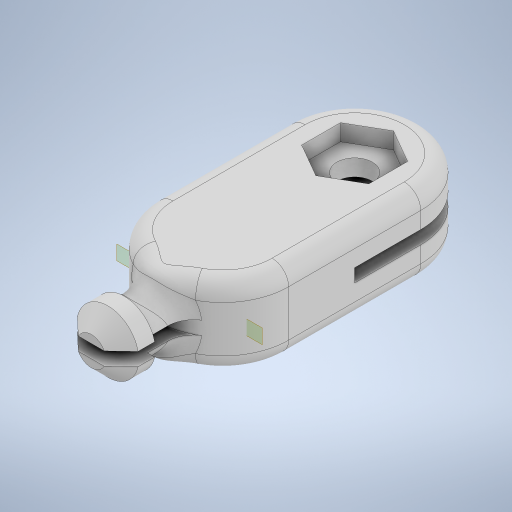
# Autodesk Inventor part: flipper_robot_v2_flipper_adapter
Saved by Autodesk Inventor 2023.1 (Build 271208000, 208)
## iProperties
Created: 2025-10-23
Part Number: flipper_robot_v2_flipper_adapter
Material: Generic
Document SubType Name: Modeling
Designer: Lars
Density: 1 g/cm^3
Appearance: Default
Author: Lars
Autodesk Inventor part; units mm, degrees
ref_plane "YZ Plane" through (0, 0, 0) normal (1, 0, 0) x (0, 1, 0)
ref_plane "XZ Plane" through (0, 0, 0) normal (0, 1, 0) x (-1, 0, 0)
ref_plane "XY Plane" through (0, 0, 0) normal (0, 0, 1) x (1, 0, 0)
sketch "Sketch1" plane through (0, 0, 0) normal (0, 1, 0) x (-1, 0, 0)
  line L0 (0, 4) -> (0, -4) construction
  line L1 (-4, 4) -> (-4, -4)
  line L2 (4, -4) -> (4, 4)
  arc A0 (4, 4) -> (-4, 4) centre (0, 4) ccw
  arc A1 (-4, -4) -> (4, -4) centre (0, -4) ccw
  circle A2 centre (0, -4) radius 1.075
  point P0 (0, 0)
  dimension "d0" = 4
  dimension "d1" = 8
  dimension "d2" = 2.15
  constraints: 8 end point, 4 point on circle, 4 tangent, 3 centre point, 1 coincident, 1 midpoint, 1 parallel, 1 vertical
  measures "d0" distance of point (0, 0) L0.end
  measures "d1" diameter of A1
  measures "d2" diameter of A2
extrude "Extrusion1" add sketch "Sketch1" along normal blind 2
sketch "Sketch2" plane through (0, 2, 0) normal (0, 1, 0) x (1, 0, 0)
  line L0 (-4, 4) -> (-4, -4) projected
  arc A0 (-4, -4) -> (4, -4) centre (0, -4) ccw projected
  line L1 (4, -4) -> (4, 4) projected
  line L2 (-4, 0) -> (4, 0)
  line L3 (0, 4) -> (0, -4) construction
  line L4 (-4, 0) -> (-4, -4)
  line L5 (4, -4) -> (4, 0)
  arc A1 (-4, -4) -> (4, -4) centre (0, -4) ccw
  point P0 (0, 0)
  constraints: 10 end point, 3 midpoint, 2 point on circle, 2 tangent, 1 centre point, 1 concentric, 1 parallel, 1 perpendicular
extrude "Extrusion2" add sketch "Sketch2" along normal blind 0.8
sketch "Sketch3" plane through (0, 2.8, 0) normal (0, 1, 0) x (1, 0, 0)
  line L0 (0, -4) -> (0, 4) construction
  line L1 (-4, -4) -> (-4, 4)
  line L2 (4, 4) -> (4, -4)
  arc A0 (-4, -4) -> (4, -4) centre (0, -4) ccw
  arc A1 (4, 4) -> (-4, 4) centre (0, 4) ccw
  circle A2 centre (0, 4) radius 1.075 projected
  circle A3 centre (0, 4) radius 1.075
  point P0 (0, 0)
  dimension "d7" = 4
  constraints: 8 end point, 4 point on circle, 4 tangent, 3 centre point, 1 coincident, 1 midpoint, 1 parallel, 1 vertical
  measures "d7" distance of point (0, 0) L0.end
extrude "Extrusion3" add sketch "Sketch3" along normal blind 2
ref_plane "Work Plane1" through (4, 2, 6) normal (0, 0, -1) x (-1, 0, 0)
sketch "Sketch4" plane through (4, 2, 6) normal (0, 0, -1) x (-1, 0, 0)
  line L0 (4, -2) -> (4, 2.8) construction
  line L1 (2.925, 2.8) -> (5.075, 2.8) projected
  line L2 (8, 0) -> (8, 0.8) projected
  line L3 (8, 0.4) -> (0, 0.4) construction
  circle A0 centre (4, 0.4) radius 2.4 construction
  line L4 (8, 2.8) -> (0, 2.8) projected
  line L5 (5.45, 0.8) -> (2.55, 0.8)
  line L6 (2.55, 0.8) -> (2.55, 0)
  line L7 (2.55, 0) -> (5.45, 0)
  line L8 (5.45, 0) -> (5.45, 0.8)
  circle A1 centre (4, 0.4) radius 1.45
  point P0 (5.45, 0.4)
  point P1 (2.55, 0.4)
  point P2 (2.0546, 1.8054)
  point P3 (5.041, 2.5625)
  point P4 (6.3869, 0.15)
  point P5 (1.6131, 0.15)
  point P6 (5.3937, 0)
  point P7 (2.6063, 0)
  point P8 (2.6063, 0.8)
  point P9 (5.3937, 0.8)
  dimension "d12" = 0.8
  dimension "d15" = 2.9
  dimension "d35" = 2.9
  constraints: 12 end point, 5 midpoint, 3 horizontal, 2 parallel, 2 point on circle, 1 centre point, 1 coincident, 1 perpendicular, 3 other
  measures "d12" distance of L6.end L5.end
  measures "d15" diameter of A1
  measures "d35" distance of L6.end L7.end
extrude "Extrusion4" add sketch "Sketch4" against normal blind 5.95 contours L5 A1 | A1 L7
sketch "Sketch6" plane through (4, 2, 11.95) normal (0, 0, 1) x (1, 0, 0)
  arc A0 (-2.1682, 0.8) -> (-5.8318, 0.8) centre (-4, 0.4) ccw
  line L0 (-5.3937, 0.8) -> (-5.8318, 0.8)
  arc A1 (-2.6063, 0.8) -> (-5.3937, 0.8) centre (-4, 0.4) ccw projected
  line L1 (-5.3937, 0.8) -> (-2.6063, 0.8) projected
  arc A2 (-2.6063, 0.8) -> (-5.3937, 0.8) centre (-4, 0.4) ccw projected
  line L2 (-5.3937, 0.8) -> (-2.6063, 0.8) projected
  line L3 (-2.6063, 0.8) -> (-2.1682, 0.8)
  line L4 (-5.8318, 0.8) -> (-5.3937, 0.8)
  point P0 (-4, -2)
  dimension "d16" = 3.75
  constraints: 6 end point, 2 collinear, 2 point on circle, 1 centre point, 1 coincident, 1 horizontal, 1 point on line
  measures "d16" diameter of A0
extrude "Extrusion5" add sketch "Sketch6" against normal blind 2 contours L3 A1 L0 A0
sketch "Sketch7" plane through (4, 2, 11.95) normal (0, 0, 1) x (1, 0, 0)
  line L0 (-2.6063, 0) -> (-5.3937, 0) projected
  arc A0 (-5.3937, 0) -> (-2.6063, 0) centre (-4, 0.4) ccw projected
  circle A1 centre (-4, 0.4) radius 1.875
  line L1 (-5.8318, 0) -> (-5.3937, 0)
  line L2 (0, 0) -> (-8, 0) projected
  line L3 (-2.6063, 0) -> (-5.3937, 0) projected
  line L4 (-2.6063, 0) -> (-2.1682, 0)
  point P0 (-4, -2)
  point P1 (-5.8318, 0.8)
  dimension "d33" = 3.75
  constraints: 4 end point, 2 point on circle, 1 centre point, 1 coincident, 1 collinear, 1 point on line
  measures "d33" diameter of A1
extrude "Extrusion6" add sketch "Sketch7" against normal blind 2 contours L2 A1 L1 A0
chamfer "Chamfer1" distance 1 angle 45 2 edges at (0, 4.275, 11.95) (0, 0.525, 11.95)
fillet "Fillet1" radius 1.5 2 edges at (0.0002, 3.85, 8) (-0.0002, 0.95, 8)
fillet "Fillet2" radius 1 12 edges at (-3.2396, 4.8, 6.3463) (0, 4.8, 8.1045) (3.2396, 4.8, 6.3463) (4, 4.8, 0) (0, 4.8, -8) (-4, 4.8, 0) (-3.2396, 0, 6.3463) (0, 0, 8.1045) (3.2396, 0, 6.3463) (4, 0, 0) (0, 0, -8) (-4, 0, 0)
sketch "Sketch8" plane through (0, 4.8, 0) normal (0, 1, 0) x (1, 0, 0)
  circle A0 centre (0, 4) radius 1.075 projected
  circle A1 centre (0, 4) radius 2.35 construction
  line L0 (0, 1.65) -> (-2.0352, 2.825)
  line L1 (-2.0352, 2.825) -> (-2.0352, 5.175)
  line L2 (-2.0352, 5.175) -> (0, 6.35)
  line L3 (0, 6.35) -> (2.0352, 5.175)
  line L4 (2.0352, 5.175) -> (2.0352, 2.825)
  line L5 (2.0352, 2.825) -> (0, 1.65)
  point P0 (0, 0)
  dimension "d28" = 4.7
  constraints: 12 end point, 2 coincident, 1 vertical alignment, 15 other
extrude "Extrusion7" cut sketch "Sketch8" against normal blind 1
equation "\"d35\" = d15"
body "Solid1"
